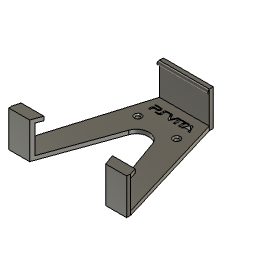
Sony PS Vita 1000 (Autodesk Fusion 360 design; units mm, degrees)
Autodesk Fusion 360 part; units mm, degrees
sketch "Top" plane through (0, 0, 0) normal (0, 0, 1) x (1, 0, 0)
  spline S0 degree 3 poles (56.9553, -10.8046) (56.9017, -10.9058) (55.889, -12.8086) (55.889, -12.8086) knots 0 0 0 0 1 1 1 1
  line L0 (55.889, -12.8086) -> (58.5008, -12.8157)
  line L1 (58.5008, -12.8157) -> (57.4264, -10.8214)
  spline S1 degree 3 poles (57.4264, -10.8214) (57.3218, -10.6112) (57.0838, -10.5593) (56.9553, -10.8046) knots 3 3 3 3 4 4 4 4
  line L2 (59.4341, -14.5484) -> (58.8429, -13.4633)
  line L3 (58.8429, -13.4633) -> (55.5299, -13.4535)
  line L4 (55.5299, -13.4535) -> (54.958, -14.5484)
  line L5 (54.958, -14.5484) -> (54.2046, -14.5484)
  spline S2 degree 3 poles (54.2046, -14.5484) (54.2047, -14.5484) (56.5526, -10.1038) (56.646, -9.9519) knots 4 4 4 4 5 5 5 5
  spline S3 degree 3 poles (56.646, -9.9519) (56.7395, -9.8001) (57.0073, -9.3204) (57.4395, -9.3438) knots 5 5 5 5 6 6 6 6
  spline S4 degree 3 poles (57.4395, -9.3438) (57.8716, -9.3671) (58.0524, -9.6962) (58.1342, -9.8363) knots 6 6 6 6 7 7 7 7
  spline S5 degree 3 poles (58.1342, -9.8363) (58.216, -9.9765) (60.6401, -14.5484) (60.6401, -14.5484) knots 7 7 7 7 8 8 8 8
  line L6 (60.6401, -14.5484) -> (59.4341, -14.5484)
  line L7 (53.1881, -10.7522) -> (53.1881, -14.5484)
  line L8 (53.1881, -14.5484) -> (52.1108, -14.5484)
  line L9 (52.1108, -14.5484) -> (52.1108, -10.6822)
  line L10 (52.1108, -10.6822) -> (52.1107, -10.0207)
  line L11 (52.1107, -10.0207) -> (51.5581, -10.0176)
  line L12 (51.5581, -10.0176) -> (50.0657, -10.0176)
  line L13 (50.0657, -10.0176) -> (50.0657, -9.3881)
  line L14 (50.0657, -9.3881) -> (51.8939, -9.3881)
  spline S6 degree 3 poles (51.8939, -9.3881) (52.3545, -9.3881) (55.241, -9.3846) (55.2411, -9.3846) knots 8 8 8 8 9 9 9 9
  line L15 (55.2411, -9.3846) -> (55.2362, -10.0214)
  line L16 (55.2362, -10.0214) -> (53.1722, -10.0171)
  line L17 (53.1722, -10.0171) -> (53.1881, -10.7522)
  line L18 (49.365, -14.5484) -> (48.2695, -14.5484)
  line L19 (48.2695, -14.5484) -> (48.2695, -9.3872)
  line L20 (48.2695, -9.3872) -> (49.365, -9.3872)
  line L21 (49.365, -9.3872) -> (49.365, -14.5484)
  spline S7 degree 3 poles (45.145, -13.9406) (45.0517, -14.0921) (44.7843, -14.5709) (44.353, -14.5476) knots 0 0 0 0 1 1 1 1
  spline S8 degree 3 poles (44.353, -14.5476) (43.9216, -14.5242) (43.7413, -14.1959) (43.6596, -14.056) knots 1 1 1 1 2 2 2 2
  spline S9 degree 3 poles (43.6596, -14.056) (43.5781, -13.9162) (41.1585, -9.353) (41.1585, -9.353) knots 2 2 2 2 3 3 3 3
  line L22 (41.1585, -9.353) -> (42.3622, -9.353)
  line L23 (42.3622, -9.353) -> (44.366, -13.0728)
  spline S10 degree 3 poles (44.366, -13.0728) (44.4705, -13.2827) (44.708, -13.3344) (44.8362, -13.0895) knots 5 5 5 5 6 6 6 6
  spline S11 degree 3 poles (44.8362, -13.0895) (44.9412, -12.8913) (46.8296, -9.353) (46.8297, -9.353) knots 6 6 6 6 7 7 7 7
  line L24 (46.8297, -9.353) -> (47.5815, -9.353)
  spline S12 degree 3 poles (47.5815, -9.353) (47.5815, -9.353) (45.2382, -13.7891) (45.145, -13.9406) knots 8 8 8 8 9 9 9 9
  line L25 (40.6794, -10.0187) -> (38.6896, -10.0187)
  spline S13 degree 3 poles (38.6896, -10.0187) (38.1521, -9.9954) (38.0448, -10.4356) (38.0448, -10.7826) knots 1 1 1 1 2 2 2 2
  line L26 (38.0448, -10.7826) -> (38.0448, -13.1454)
  spline S14 degree 3 poles (38.0448, -13.1454) (38.0448, -14.0094) (37.6559, -14.5484) (36.5778, -14.5484) knots 3 3 3 3 4 4 4 4
  line L27 (36.5778, -14.5484) -> (34.262, -14.5484)
  line L28 (34.262, -14.5484) -> (34.262, -13.9096)
  line L29 (34.262, -13.9096) -> (36.2825, -13.9096)
  spline S15 degree 3 poles (36.2825, -13.9096) (36.696, -13.9096) (36.943, -13.5737) (36.943, -13.1454) knots 7 7 7 7 8 8 8 8
  line L30 (36.943, -13.1454) -> (36.943, -10.7826)
  spline S16 degree 3 poles (36.943, -10.7826) (36.943, -10.0295) (37.3089, -9.3797) (38.3795, -9.3797) knots 9 9 9 9 10 10 10 10
  line L31 (38.3795, -9.3797) -> (40.6794, -9.3797)
  line L32 (40.6794, -9.3797) -> (40.6794, -10.0187)
  spline S17 degree 3 poles (31.0205, -12.2372) (30.6808, -12.2372) (30.4298, -12.4957) (30.4298, -12.9387) knots 0 0 0 0 1 1 1 1
  line L33 (30.4298, -12.9387) -> (30.4298, -14.5484)
  line L34 (30.4298, -14.5484) -> (29.3599, -14.5484)
  line L35 (29.3599, -14.5484) -> (29.3599, -12.9978)
  spline S18 degree 3 poles (29.3599, -12.9978) (29.3599, -12.1265) (29.9063, -11.5394) (30.6816, -11.5394) knots 4 4 4 4 5 5 5 5
  line L36 (30.6816, -11.5394) -> (33.1885, -11.5394)
  spline S19 degree 3 poles (33.1885, -11.5394) (33.8034, -11.5161) (33.95, -11.2109) (33.95, -10.7679) (33.95, -10.4282) (33.78, -9.9646) (33.1885, -10.0113) knots 6 6 6 6 7 7 7 8 8 8 8
  line L37 (33.1885, -10.0113) -> (29.3599, -10.0113)
  line L38 (29.3599, -10.0113) -> (29.3599, -9.3723)
  line L39 (29.3599, -9.3723) -> (33.4987, -9.3723)
  spline S20 degree 3 poles (33.4987, -9.3723) (34.5841, -9.3723) (35.0124, -9.9999) (35.0124, -10.7679) (35.0124, -11.6392) (34.5841, -12.2372) (33.4987, -12.2372) knots 11 11 11 11 12 12 12 13 13 13 13
  line L40 (33.4987, -12.2372) -> (31.0205, -12.2372)
  line L41 (64, -3) -> (64, 0)
  line L42 (64, 0) -> (26, 0)
  line L43 (26, 0) -> (26, -3)
  line L44 (26, -3) -> (0, -89)
  line L45 (0, -89) -> (0, -92)
  line L46 (0, -92) -> (16, -92)
  line L47 (16, -92) -> (35.9939, -36.4259)
  spline S21 degree 3 poles (35.9939, -36.4259) (39.0309, -27.9844) (50.9691, -27.9844) (54.0061, -36.4259) knots 7 7 7 7 8 8 8 8
  line L48 (54.0061, -36.4259) -> (74, -92)
  line L49 (74, -92) -> (90, -92)
  line L50 (90, -92) -> (90, -89)
  line L51 (90, -89) -> (64, -3)
extrude "Extrude1" add sketch "Top" along normal blind 27.5 contours L41 L42 L43 L44 L45 L46 L47 S21 L48 L49 L50 L51
sketch "RightSideCut" plane through (0, 0, 0) normal (1, 0, 0) x (0, 1, 0)
  line L0 (-92, 32.5) -> (-92, 27.5)
  line L1 (-92, 27.5) -> (-84, 27.5)
  line L2 (-84, 27.5) -> (-84, 24.5)
  line L3 (-84, 24.5) -> (-89, 24.5)
  line L4 (-89, 24.5) -> (-89, 3)
  line L5 (-89, 3) -> (-3, 3)
  line L6 (-3, 3) -> (-3, 24.5)
  spline S0 degree 3 poles (-3, 24.5) (-3.8284, 24.5) (-4.5, 25.1716) (-4.5, 26) (-4.5, 26.8284) (-3.8284, 27.5) (-3, 27.5) knots 7 7 7 7 8 8 8 9 9 9 9
  line L7 (-3, 27.5) -> (0, 27.5)
  line L8 (0, 27.5) -> (0, 32.5)
  line L9 (0, 32.5) -> (-92, 32.5)
extrude "Extrude2" cut sketch "RightSideCut" along normal blind 90
hole "Hole1" at (30.2041, -23.6497, 3) direction (0, 0, -1) diameter 3.5 depth 3 tip angle 118 countersink diameter 5.5 countersink angle 90
hole "Hole2" at (59.7962, -23.65, 3) direction (0, 0, -1) diameter 3.5 depth 3 tip angle 118 countersink diameter 5.5 countersink angle 90
